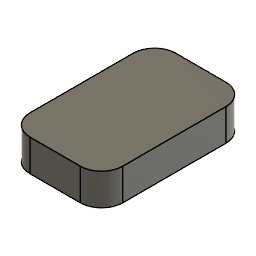
RobotDog_Final (Autodesk Fusion 360 archive; units mm, degrees)
design "Foot"
part number: 2026-07-09-18-11-10-596
Autodesk Fusion 360 part; units mm, degrees
sketch "Sketch1" plane through (0, 0, 0) normal (0, 1, 0) x (1, 0, 0)
  line L0 (-99.8337, 61.2286) -> (-64.8337, 61.2286)
  line L1 (-64.8337, 61.2286) -> (-64.8337, 116.2286)
  line L2 (-64.8337, 116.2286) -> (-99.8337, 116.2286)
  line L3 (-99.8337, 116.2286) -> (-99.8337, 61.2286)
  line L4 (-99.8337, 61.2286) -> (-64.8337, 116.2286) construction
  line L5 (-64.8337, 61.2286) -> (-99.8337, 116.2286) construction
  point P0 (-82.3337, 88.7286)
  dimension "d1" = 35
  dimension "d2" = 55
  constraint horizontal L0
  constraint perpendicular L0 L1
  constraint parallel L0 L2
  constraint parallel L1 L3
  constraint coincident L4 P0
  constraint coincident L5 P0
  measures "d1" distance of L1.end L2.end
  measures "d2" distance of L0.end L1.end
extrude "Extrude1" add sketch "Sketch1" along normal blind 12
fillet "Fillet1" radius 8 4 edges at (-99.8337, 6, -116.2286) (-64.8337, 6, -116.2286) (-99.8337, 6, -61.2286) (-64.8337, 6, -61.2286)

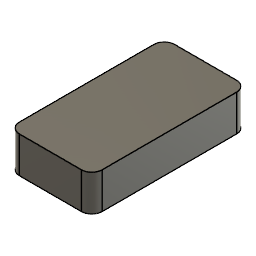
design "body"
part number: 2026-07-09-17-18-24-352
Autodesk Fusion 360 part; units mm, degrees
sketch "Sketch1" plane through (0, 0, 0) normal (0, 1, 0) x (1, 0, 0)
  line L0 (-80, 150) -> (80, 150)
  line L1 (80, 150) -> (80, -150)
  line L2 (80, -150) -> (-80, -150)
  line L3 (-80, -150) -> (-80, 150)
  line L4 (-80, 150) -> (80, -150) construction
  line L5 (80, 150) -> (-80, -150) construction
  dimension "d1" = 160
  dimension "d2" = 300
  constraint horizontal L0
  constraint perpendicular L0 L1
  constraint parallel L0 L2
  constraint parallel L1 L3
  constraint coincident L4 origin
  constraint coincident L5 origin
  measures "d1" distance of L1.end L2.end
  measures "d2" distance of L0.end L1.end
extrude "Extrude1" add sketch "Sketch1" along normal blind 70
fillet "Fillet1" radius 20 4 edges at (80, 35, 150) (-80, 35, 150) (80, 35, -150) (-80, 35, -150)

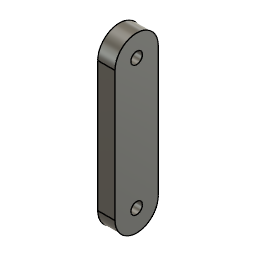
design "Upper_Leg"
part number: 2026-07-09-17-25-33-215
Autodesk Fusion 360 part; units mm, degrees
sketch "Sketch1" plane through (0, 0, 0) normal (1, 0, 0) x (0, 0, -1)
  line L0 (-11.8042, 4.5566) -> (-41.8042, 4.5566)
  line L1 (-41.8042, 4.5566) -> (-41.8042, 124.5566)
  line L2 (-41.8042, 124.5566) -> (-11.8042, 124.5566)
  line L3 (-11.8042, 124.5566) -> (-11.8042, 4.5566)
  line L4 (-11.8042, 4.5566) -> (-41.8042, 124.5566) construction
  line L5 (-41.8042, 4.5566) -> (-11.8042, 124.5566) construction
  point P0 (-26.8042, 64.5566)
  dimension "d1" = 30
  dimension "d2" = 120
  constraint horizontal L0
  constraint perpendicular L0 L1
  constraint parallel L0 L2
  constraint parallel L1 L3
  constraint coincident L4 P0
  constraint coincident L5 P0
  measures "d1" distance of L1.end L2.end
  measures "d2" distance of L0.end L1.end
extrude "Extrude1" add sketch "Sketch1" along normal blind 12
fillet "Fillet1" radius 15 4 edges at (6, 124.5566, 41.8042) (6, 124.5566, 11.8042) (6, 4.5566, 41.8042) (6, 4.5566, 11.8042)
sketch "Sketch2" plane through (12, 0, 0) normal (1, 0, 0) x (0, 0, -1)
  arc A0 (-41.8042, 19.5566) -> (-11.8042, 19.5566) centre (-26.8042, 19.5566) ccw
  line L0 (-11.8042, 19.5566) -> (-11.8042, 109.5566)
  arc A1 (-11.8042, 109.5566) -> (-41.8042, 109.5566) centre (-26.8042, 109.5566) ccw
  line L1 (-41.8042, 109.5566) -> (-41.8042, 19.5566)
  circle A2 centre (-26.8042, 19.5566) radius 4
  circle A3 centre (-26.8042, 109.5566) radius 4
  dimension "d7" = 8
  dimension "d8" = 8
  constraint concentric A0 A2
  constraint concentric A1 A3
  measures "d7" diameter of A2
  measures "d8" diameter of A3
extrude "Extrude2" cut sketch "Sketch2" against normal through all contours A2 | A3

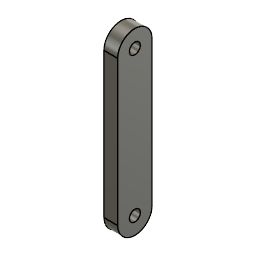
design "Lower_Leg"
part number: 2026-07-09-17-42-01-885
Autodesk Fusion 360 part; units mm, degrees
sketch "Sketch1" plane through (0, 0, 0) normal (1, 0, 0) x (0, 0, -1)
  line L0 (-17.5, 45) -> (-42.5, 45)
  line L1 (-42.5, 45) -> (-42.5, 175)
  line L2 (-42.5, 175) -> (-17.5, 175)
  line L3 (-17.5, 175) -> (-17.5, 45)
  line L4 (-17.5, 45) -> (-42.5, 175) construction
  line L5 (-42.5, 45) -> (-17.5, 175) construction
  point P0 (-30, 110)
  dimension "d1" = 25
  dimension "d2" = 130
  constraint horizontal L0
  constraint perpendicular L0 L1
  constraint parallel L0 L2
  constraint parallel L1 L3
  constraint coincident L4 P0
  constraint coincident L5 P0
  measures "d1" distance of L1.end L2.end
  measures "d2" distance of L0.end L1.end
extrude "Extrude1" add sketch "Sketch1" along normal blind 10
fillet "Fillet1" radius 12.5 4 edges at (5, 175, 42.5) (5, 45, 42.5) (5, 45, 17.5) (5, 175, 17.5)
sketch "Sketch2" plane through (10, 0, 0) normal (1, 0, 0) x (0, 0, -1)
  arc A0 (-17.5, 162.5) -> (-42.5, 162.5) centre (-30, 162.5) ccw
  line L0 (-42.5, 162.5) -> (-42.5, 57.5)
  arc A1 (-42.5, 57.5) -> (-17.5, 57.5) centre (-30, 57.5) ccw
  line L1 (-17.5, 57.5) -> (-17.5, 162.5)
  circle A2 centre (-30, 162.5) radius 4
  circle A3 centre (-30, 57.5) radius 4
  dimension "d7" = 8
  dimension "d8" = 8
  constraint concentric A0 A2
  constraint concentric A1 A3
  measures "d7" diameter of A2
  measures "d8" diameter of A3
extrude "Extrude2" cut sketch "Sketch2" against normal through all contours A2 | A3
